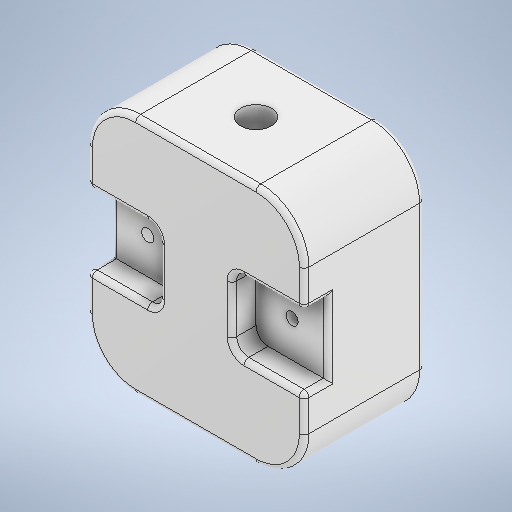
# Autodesk Inventor part: Madeira
Saved by Autodesk Inventor 2025 (Build 290162010, 162A)
## iProperties
Created: 2024-06-10
Part Number: Madeira
Material: PBT Plastic
Document SubType Name: Modeling
Designer: bryan
Density: 1.31 g/cm^3
Appearance: Smooth - White
Mass: 525.828 g
Surface Area: 396.557 cm^2
Volume: 401.396 cm^3
Author: bryan
Autodesk Inventor part; units mm, degrees
ref_plane "YZ Plane" through (0, 0, 0) normal (1, 0, 0) x (0, 1, 0)
ref_plane "XZ Plane" through (0, 0, 0) normal (0, 1, 0) x (-1, 0, 0)
ref_plane "XY Plane" through (0, 0, 0) normal (0, 0, 1) x (1, 0, 0)
sketch "Sketch1" plane through (0, 0, 0) normal (0, 1, 0) x (-1, 0, 0)
  line L0 (0, 0) -> (100, 0)
  line L1 (100, 0) -> (100, -50)
  line L2 (100, -50) -> (0, -50)
  line L3 (0, -50) -> (0, 0)
  dimension "d0" = 100
  dimension "d1" = 50
  constraints: 8 end point, 2 parallel, 1 horizontal, 1 perpendicular
  measures "d0" distance of L1.end L2.end
  measures "d1" distance of L0.end L1.end
extrude "Extrusion1" add sketch "Sketch1" along normal blind 250
sketch "Sketch5" plane through (0, 0, -50) normal (0, 0, -1) x (-1, 0, 0)
  line L0 (0, 250) -> (100, 250) projected
  line L1 (100, 0) -> (100, 250) projected
  circle A0 centre (50, 125) radius 5
  point P0 (0, 0)
  dimension "d85" = 10
  constraints: 1 centre point
  measures "d85" diameter of A0
extrude "Extrusion5" cut sketch "Sketch5" against normal through all
sketch "Sketch6" plane through (0, 0, 0) normal (0, -1, 0) x (1, 0, 0)
  line L0 (-100, 0) -> (0, 0) projected
  line L1 (0, -50) -> (-15, -50)
  line L2 (-15, -50) -> (-15, 0)
  line L3 (-15, 0) -> (0, 0)
  line L4 (0, 0) -> (0, -50)
  line L5 (-100, -50) -> (-100, 0) projected
  line L6 (-100, -50) -> (-85, -50)
  line L7 (-85, -50) -> (-85, 0)
  line L8 (-85, 0) -> (-100, 0)
  line L9 (-100, 0) -> (-100, -50)
  dimension "d18" = 15
  dimension "d19" = 15
  constraints: 16 end point, 4 parallel, 2 horizontal, 2 perpendicular, 2 point on line
  measures "d18" distance of L2.end L3.end
  measures "d19" distance of L8.end L7.end
extrude "Extrusion6" cut sketch "Sketch6" against normal through all
sketch "Sketch7" plane through (0, 0, 0) normal (0, -1, 0) x (1, 0, 0)
  line L0 (-15, -50) -> (-85, -50) projected
  line L1 (-85, 0) -> (-15, 0) projected
  line L2 (-15, -50) -> (-85, -50)
  line L3 (-85, -50) -> (-85, 0)
  line L4 (-85, 0) -> (-15, 0)
  line L5 (-15, 0) -> (-15, -50)
  point P0 (0, 0)
  constraints: 8 end point, 2 parallel, 1 horizontal, 1 perpendicular
extrude "Extrusion7" cut sketch "Sketch7" against normal blind 50
sketch "Sketch8" plane through (0, 250, 0) normal (0, 1, 0) x (1, 0, 0)
  line L0 (-15, 50) -> (-85, 50) projected
  line L1 (-15, 0) -> (-15, 50) projected
  line L2 (-85, 50) -> (-15, 50)
  line L3 (-15, 50) -> (-15, 0)
  line L4 (-15, 0) -> (-85, 0)
  line L5 (-85, 0) -> (-85, 50)
  point P0 (0, 0)
  constraints: 8 end point, 2 parallel, 1 horizontal, 1 perpendicular
extrude "Extrusion8" cut sketch "Sketch8" against normal blind 50
sketch "Sketch14" plane through (0, 200, 0) normal (0, 1, 0) x (1, 0, 0)
  point P0 (0, 0)
sketch "Sketch15" plane through (0, 200, 0) normal (0, 1, 0) x (1, 0, 0)
  line L0 (-15, 50) -> (-15, 0) projected
  line L1 (-85, 0) -> (-85, 50) projected
  line L2 (-15, 50) -> (-85, 50)
  line L3 (-85, 50) -> (-85, 45)
  line L4 (-85, 45) -> (-15, 45)
  line L5 (-15, 45) -> (-15, 50)
  line L6 (-15, 0) -> (-85, 0)
  line L7 (-85, 0) -> (-85, 5)
  line L8 (-85, 5) -> (-15, 5)
  line L9 (-15, 5) -> (-15, 0)
  point P0 (0, 0)
  dimension "d46" = 5
  dimension "d47" = 5
  constraints: 16 end point, 4 parallel, 2 horizontal, 2 perpendicular, 2 point on line
  measures "d46" distance of L3.end L2.end
  measures "d47" distance of L6.end L7.end
extrude "Extrusion13" cut sketch "Sketch15" against normal through all contours L0 L4 L1 L2 | L0 L6 L1 L8
sketch "Sketch16" plane through (-85, 50, -45) normal (-1, 0, 0) x (0, 0, 1)
  line L0 (45, 92.6169) -> (35, 92.6169)
  line L1 (35, 92.6169) -> (35, 57.3831)
  line L2 (35, 57.3831) -> (45, 57.3831)
  line L3 (45, 57.3831) -> (45, 92.6169)
  line L4 (40, 150) -> (40, 0) projected
  line L5 (45, 92.6169) -> (35, 57.3831) construction
  line L6 (35, 92.6169) -> (45, 57.3831) construction
  line L7 (40, 92.6169) -> (40, 57.3831)
  point P0 (45, -50)
  point P1 (40, 75)
  dimension "d50" = 10
  constraints: 14 end point, 5 midpoint, 2 parallel, 2 point on line, 1 horizontal, 1 perpendicular
  measures "d50" distance of L2.end L1.end
extrude "Extrusion14" add sketch "Sketch16" along normal blind 34.5 contours L4 L2 L1 L0
sketch "Sketch17" plane through (-85, 200, -5) normal (0, 0, 1) x (1, 0, 0)
  line L0 (-34.5, -92.6169) -> (-34.5, -57.3831) projected
  line L1 (-34.5, -75) -> (-29.5, -75)
  circle A0 centre (-29.5, -75) radius 2.5
  point P0 (85, -200)
  dimension "d53" = 5
  dimension "d54" = 5
  constraints: 2 end point, 1 centre point, 1 coincident, 1 horizontal, 1 midpoint
  measures "d53" distance of L1.start L1.end
  measures "d54" diameter of A0
extrude "Extrusion15" cut sketch "Sketch17" against normal through all
thread "Thread1" size "M5x0.8" class "6H" standard "ANSI Metric M Profile" full length
sketch "Sketch19" plane through (-119.5, 50, -45) normal (-1, 0, 0) x (0, 0, 1)
  line L0 (40, 57.3831) -> (40, 92.6169) projected
  line L1 (40, 57.3831) -> (35, 57.3831) projected
  line L2 (40, 92.6169) -> (35, 92.6169)
  line L3 (35, 92.6169) -> (35, 57.3831)
  line L4 (35, 57.3831) -> (40, 57.3831)
  line L5 (40, 57.3831) -> (40, 92.6169)
  point P0 (45, -50)
  constraints: 8 end point, 2 parallel, 1 horizontal, 1 perpendicular
extrude "Extrusion17" add sketch "Sketch19" along normal blind 32
sketch "Sketch20" plane through (-85, 200, -5) normal (0, 0, 1) x (1, 0, 0)
  line L0 (-66.5, -92.6169) -> (-66.5, -57.3831) projected
  circle A0 centre (-61.5, -75) radius 2.5
  point P0 (85, -200)
  dimension "d73" = 5
  constraints: 1 centre point
  measures "d73" diameter of A0
extrude "Extrusion18" cut sketch "Sketch20" against normal blind 32
thread "Thread2" size "M5x0.8" class "6H" standard "ANSI Metric M Profile" full length
sketch "Sketch21" plane through (0, 50, 0) normal (0, -1, 0) x (1, 0, 0)
  line L0 (-15, -5) -> (-85, -5) projected
  line L1 (-15, -5) -> (-15, -45) projected
  circle A0 centre (-50, -25) radius 7.5
  point P0 (0, 0)
  dimension "d86" = 15
  constraints: 1 centre point
  measures "d86" diameter of A0
extrude "Extrusion19" cut sketch "Sketch21" against normal blind 55
sketch "Sketch22" plane through (0, 200, 0) normal (0, 1, 0) x (1, 0, 0)
  circle A0 centre (-50, 25) radius 7.5
  point P0 (0, 0)
  dimension "d87" = 15
  constraints: 1 centre point, 1 coincident
  measures "d87" diameter of A0
extrude "Extrusion20" cut sketch "Sketch22" against normal blind 55
fillet "Fillet1" radius 10 4 edges at (-85, 200, -25) (-15, 200, -25) (-85, 50, -25) (-15, 50, -25)
sketch "Sketch23" plane through (-85, 107.3831, -10) normal (0, 0, -1) x (-1, 0, 0)
  circle A0 centre (61.5, 17.6169) radius 2.5 projected
  circle A1 centre (61.5, 17.6169) radius 2.5 projected
  line L0 (66.5, 35.2339) -> (66.5, 0) projected
  circle A2 centre (29.5, 17.6169) radius 2.5 projected
  line L1 (0, 0) -> (66.5, 0) projected
  circle A3 centre (61.5, 17.6169) radius 2.5 projected
  circle A4 centre (29.5, 17.6169) radius 2.5 projected
  line L2 (0, 0) -> (0, 35.2339) projected
  line L3 (0, 0) -> (66.5, 0) projected
  line L4 (66.5, 35.2339) -> (66.5, 0) projected
  line L5 (0, 35.2339) -> (66.5, 35.2339) projected
  point P0 (-85, -107.3831)
extrude "Extrusion21" add sketch "Sketch23" along normal blind 5
fillet "Fillet2" radius 30 2 edges at (-85, 142.6169, -10) (-85, 107.3831, -10)
fillet "Fillet3" radius 10 2 edges at (-151.5, 107.3831, -10) (-151.5, 142.6169, -10)
fillet "Fillet4" radius 20 1 edges at (-85, 125, -15)
sketch "Sketch25" plane through (-151.5, 50, -45) normal (-1, 0, 0) x (0, 0, 1)
  line L0 (30, 92.6169) -> (40, 92.6169) projected
  line L1 (30, 92.6169) -> (40, 92.6169)
  line L2 (40, 92.6169) -> (40, 57.3831)
  line L3 (40, 57.3831) -> (30, 57.3831)
  line L4 (30, 57.3831) -> (30, 92.6169)
  point P0 (45, -50)
  constraints: 8 end point, 2 parallel, 1 horizontal, 1 perpendicular
extrude "Extrusion22" add sketch "Sketch25" against normal blind 10
fillet "Fillet5" radius 10 2 edges at (-151.5, 107.3831, -10) (-151.5, 142.6169, -10)
sketch "Sketch26" plane through (-75, 200, -5) normal (0, 0, 1) x (1, 0, 0)
  circle A0 centre (-71.5, -75) radius 2.5
  circle A1 centre (-39.5, -75) radius 2.5 projected
  point P0 (75, -200)
  dimension "d91" = 5
  dimension "d92" = 32
  constraints: 1 centre point
  measures "d91" diameter of A0
  measures "d92" distance of A1.centre A0.centre
extrude "Extrusion23" cut sketch "Sketch26" against normal blind 10 contours A0
sketch "Sketch27" plane through (0, 200, 0) normal (0, 1, 0) x (1, 0, 0)
  line L0 (-85, 45) -> (-85, 5) projected
  line L1 (-5.7432, 0) -> (-85, 0)
  line L2 (-85, 0) -> (-85, 45)
  line L3 (-85, 45) -> (-5.7432, 45)
  line L4 (-5.7432, 45) -> (-5.7432, 0)
  line L5 (-85, 0) -> (-209.0524, 0)
  line L6 (-209.0524, 0) -> (-209.0524, 63.2581)
  line L7 (-209.0524, 63.2581) -> (-85, 63.2581)
  line L8 (-85, 63.2581) -> (-85, 0)
  point P0 (0, 0)
  constraints: 16 end point, 4 parallel, 2 horizontal, 2 perpendicular
extrude "Extrusion24" cut sketch "Sketch27" against normal up to surface (150 mm away) contours L0 L2 L5 L6 L7 L8
sketch "Sketch28" plane through (-75, 200, -5) normal (0, 0, 1) x (1, 0, 0)
  line L0 (-10, -140) -> (-10, -10) projected
  arc A0 (-10, -140) -> (0, -150) centre (0, -140) ccw projected
  line L1 (50, -150) -> (0, -150) projected
  arc A1 (50, -150) -> (60, -140) centre (50, -140) ccw projected
  line L2 (60, -10) -> (60, -140) projected
  arc A2 (60, -10) -> (50, 0) centre (50, -10) ccw projected
  line L3 (0, 0) -> (50, 0) projected
  arc A3 (0, 0) -> (-10, -10) centre (0, -10) ccw projected
  circle A4 centre (25, -75) radius 5 projected
  line L4 (32.5, -95) -> (17.5, -95) projected
  arc A5 (50, -150) -> (60, -140) centre (50, -140) ccw projected
  line L5 (0, -150) -> (50, -150) projected
  arc A6 (-10, -140) -> (0, -150) centre (0, -140) ccw projected
  line L6 (-10, -10) -> (-10, -140) projected
  arc A7 (0, 0) -> (-10, -10) centre (0, -10) ccw projected
  line L7 (50, 0) -> (0, 0) projected
  arc A8 (60, -10) -> (50, 0) centre (50, -10) ccw projected
  line L8 (60, -140) -> (60, -10) projected
  circle A9 centre (25, -75) radius 5 projected
  point P0 (75, -200)
extrude "Extrusion25" add sketch "Sketch28" along normal blind 5
sketch "Sketch29" plane through (-25, 200, -45) normal (0, 0, -1) x (-1, 0, 0)
  arc A0 (-10, -140) -> (0, -150) centre (0, -140) ccw projected
  line L0 (50, -150) -> (0, -150) projected
  arc A1 (50, -150) -> (60, -140) centre (50, -140) ccw projected
  line L1 (60, -10) -> (60, -140) projected
  arc A2 (60, -10) -> (50, 0) centre (50, -10) ccw projected
  line L2 (0, 0) -> (50, 0) projected
  arc A3 (0, 0) -> (-10, -10) centre (0, -10) ccw projected
  line L3 (-10, -140) -> (-10, -10) projected
  circle A4 centre (25, -75) radius 5 projected
  point P0 (-25, -200)
extrude "Extrusion26" add sketch "Sketch29" along normal blind 5
sketch "Sketch37" plane through (-75, 200, 0) normal (0, 0, 1) x (1, 0, 0)
  point P0 (75, -200)
sketch "Sketch38" plane through (0, 50, 0) normal (0, -1, 0) x (1, 0, 0)
  line L0 (-85, 0) -> (-15, 0)
  line L1 (-15, 0) -> (-15, -50)
  line L2 (-15, -50) -> (-85, -50)
  line L3 (-85, -50) -> (-85, 0)
  circle A0 centre (-50, -25) radius 7.5 projected
  line L4 (-85, 0) -> (-15, -50) construction
  line L5 (-15, 0) -> (-85, -50) construction
  point P0 (0, 0)
  constraints: 12 end point, 2 midpoint, 2 parallel, 1 perpendicular
extrude "Extrusion32" cut sketch "Sketch38" against normal blind 10
sketch "Sketch39" plane through (0, 200, 0) normal (0, 1, 0) x (1, 0, 0)
  line L0 (-15, 0) -> (-85, 0)
  line L1 (-85, 0) -> (-85, 50)
  line L2 (-85, 50) -> (-15, 50)
  line L3 (-15, 50) -> (-15, 0)
  circle A0 centre (-50, 25) radius 7.5 projected
  line L4 (-15, 0) -> (-85, 50) construction
  line L5 (-85, 0) -> (-15, 50) construction
  point P0 (0, 0)
  constraints: 12 end point, 2 midpoint, 2 parallel, 1 perpendicular
extrude "Extrusion33" cut sketch "Sketch39" against normal blind 10
sketch "Sketch40" plane through (-85, 60, -50) normal (-1, 0, 0) x (0, 0, 1)
  line L0 (50, 130) -> (0, 130) projected
  line L1 (50, 0) -> (0, 0) projected
  line L2 (50, 130) -> (0, 130)
  line L3 (0, 130) -> (0, 0)
  line L4 (0, 0) -> (50, 0)
  line L5 (50, 0) -> (50, 130)
  point P0 (50, -60)
  constraints: 8 end point, 2 parallel, 1 horizontal, 1 perpendicular
extrude "Extrusion34" add sketch "Sketch40" along normal blind 10
sketch "Sketch41" plane through (-15, 60, 0) normal (1, 0, 0) x (0, 0, -1)
  line L0 (0, 130) -> (50, 130) projected
  line L1 (0, 0) -> (0, 130) projected
  line L2 (50, 130) -> (0, 130)
  line L3 (0, 130) -> (0, 0)
  line L4 (0, 0) -> (50, 0)
  line L5 (50, 0) -> (50, 130)
  point P0 (0, -60)
  constraints: 8 end point, 2 parallel, 1 horizontal, 1 perpendicular
extrude "Extrusion35" add sketch "Sketch41" along normal blind 10
sketch "Sketch42" plane through (-75, 200, 0) normal (0, 0, 1) x (1, 0, 0)
  line L0 (-20, -10) -> (-20, -140) projected
  line L1 (-20, -95) -> (-20, -55)
  line L2 (10, -75) -> (10, -90)
  line L3 (10, -75) -> (10, -60)
  line L4 (10, -60) -> (-20, -60)
  line L5 (10, -90) -> (-20, -90)
  line L6 (-20, -75) -> (10, -75)
  circle A0 centre (-5, -75) radius 2.5
  point P0 (75, -200)
  dimension "d144" = 5
  constraints: 12 end point, 2 midpoint, 2 perpendicular, 2 point on line, 1 centre point, 1 horizontal
  measures "d144" diameter of A0
extrude "Extrusion36" cut sketch "Sketch42" against normal blind 10 contours L4 L3 L6 A0 L0 | L6 A0 L2 L5 L0
sketch "Sketch43" plane through (-75, 200, 0) normal (0, 0, 1) x (1, 0, 0)
  line L0 (-20, -140) -> (-20, -10) projected
  point P0 (75, -200)
extrude "Extrusion37" cut sketch "Sketch42" against normal up to surface (50 mm away) contours A0 L6 | L6 A0
sketch "Sketch44" plane through (-75, 200, 0) normal (0, 0, 1) x (1, 0, 0)
  line L0 (-20, -60) -> (10, -60) projected
  line L1 (10, -90) -> (-20, -90) projected
  line L2 (10, -60) -> (10, -90) projected
  line L3 (70, -140) -> (70, -10) projected
  line L4 (70, -90) -> (40, -90)
  line L5 (40, -90) -> (40, -60)
  line L6 (40, -60) -> (70, -60)
  line L7 (70, -60) -> (70, -90)
  circle A0 centre (55, -75) radius 2.5
  point P0 (75, -200)
  dimension "d147" = 30
  dimension "d150" = 5
  constraints: 8 end point, 2 parallel, 1 centre point, 1 horizontal, 1 perpendicular, 1 point on line
  measures "d147" distance of L5.end L6.end
  measures "d150" diameter of A0
extrude "Extrusion38" cut sketch "Sketch44" against normal blind 10
extrude "Extrusion39" cut sketch "Sketch44" against normal up to surface (50 mm away) contours A0
fillet "Fillet7" radius 5 4 edges at (-35, 110, -5) (-35, 140, -5) (-65, 140, -5) (-65, 110, -5)
fillet "Fillet8" radius 2 6 edges at (-5, 110, -5) (-5, 140, -5) (-5, 125, -10) (-95, 125, -10) (-95, 140, -5) (-95, 110, -5)
sketch "Sketch45" plane through (-75, 200, 0) normal (0, 0, 1) x (1, 0, 0)
  line L0 (-20, -10) -> (-20, -140) projected
  line L1 (70, -140) -> (70, -10) projected
  line L2 (-20, -140) -> (70, -140)
  line L3 (70, -140) -> (70, -125)
  line L4 (70, -125) -> (-20, -125)
  line L5 (-20, -125) -> (-20, -140)
  line L6 (-20, -10) -> (70, -10) projected
  line L7 (-20, -10) -> (70, -10)
  line L8 (70, -10) -> (70, -25)
  line L9 (70, -25) -> (-20, -25)
  line L10 (-20, -25) -> (-20, -10)
  point P0 (75, -200)
  dimension "d158" = 15
  dimension "d159" = 15
  constraints: 16 end point, 4 parallel, 2 horizontal, 2 perpendicular, 2 point on line
  measures "d158" distance of L3.end L2.end
  measures "d159" distance of L7.end L8.end
extrude "Extrusion40" cut sketch "Sketch45" against normal up to surface (50 mm away) contours L6 L1 L9 L0 | L4 L1 L2 L0
sketch "Sketch46" plane through (-75, 200, 0) normal (0, 0, 1) x (1, 0, 0)
  circle A0 centre (25, -75) radius 5 projected
  circle A1 centre (25, -75) radius 5
  point P0 (75, -200)
  constraints: 1 centre point, 1 coincident
extrude "Extrusion41" add sketch "Sketch46" against normal up to surface (50 mm away)
sketch "Sketch47" plane through (-95, 175, 0) normal (0, 1, 0) x (1, 0, 0)
  circle A0 centre (45, 25) radius 7.5 projected
  circle A1 centre (45, 25) radius 7.5
  circle A2 centre (45, 25) radius 7.5 projected
  point P0 (95, 0)
  constraints: 1 centre point, 1 coincident
extrude "Extrusion42" cut sketch "Sketch47" against normal up to surface (100 mm away)
fillet "Fillet9" radius 20 4 edges at (-95, 175, -25) (-95, 75, -25) (-5, 75, -25) (-5, 175, -25)
fillet "Fillet10" radius 2 32 edges at (-89.1421, 80.8579, -50) (-50, 75, -50) (-10.8579, 80.8579, -50) (-5, 125, -50) (-10.8579, 169.1421, -50) (-50, 175, -50) (-89.1421, 169.1421, -50) (-95, 125, -50) (-50, 175, 0) (-10.8579, 169.1421, 0) (-5, 148.5, 0) (-5, 101.5, 0) (-5.5858, 140.5858, 0) (-18.5, 140, 0) (-33.5355, 138.5355, 0) (-35, 125, 0) (-33.5355, 111.4645, 0) (-18.5, 110, 0) (-5.5858, 109.4142, 0) (-10.8579, 80.8579, 0) (-50, 75, 0) (-89.1421, 80.8579, 0) (-95, 148.5, 0) (-95, 101.5, 0) (-94.4142, 109.4142, 0) (-81.5, 110, 0) (-66.4645, 111.4645, 0) (-65, 125, 0) (-66.4645, 138.5355, 0) (-81.5, 140, 0) (-94.4142, 140.5858, 0) (-89.1421, 169.1421, 0)
sketch "Sketch48" plane through (-75, 75, -2) normal (0, -1, 0) x (1, 0, 0)
  circle A0 centre (25, -23) radius 7.5 projected
  circle A1 centre (25, -23) radius 7.5
  point P0 (75, 2)
  constraints: 1 centre point, 1 coincident
extrude "Extrusion43" add sketch "Sketch48" against normal up to surface (100 mm away)
sketch "Sketch49" plane through (-75, 75, -2) normal (0, -1, 0) x (1, 0, 0)
  circle A0 centre (25, -23) radius 7.5 projected
  circle A1 centre (25, -23) radius 6
  point P0 (75, 2)
  dimension "d170" = 12
  constraints: 1 centre point, 1 coincident
  measures "d170" diameter of A1
extrude "Extrusion44" cut sketch "Sketch49" against normal up to surface (100 mm away) contours A1
sketch "Sketch50" plane through (-75, 75, -2) normal (0, -1, 0) x (1, 0, 0)
  circle A0 centre (25, -23) radius 6 projected
  circle A1 centre (25, -23) radius 6.4
  point P0 (75, 2)
  dimension "d173" = 12.8
  constraints: 1 centre point, 1 coincident
  measures "d173" diameter of A1
extrude "Extrusion45" cut sketch "Sketch50" against normal up to surface (100 mm away)
body "Solid1"
